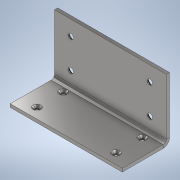
# Autodesk Inventor part: Pletina
Saved by Autodesk Inventor 2021 (Build 250183000, 183)
## iProperties
Created: 2020-10-24
Part Number: Pletina
Material: Steel, Carbon
Document SubType Name: Sheet Metal
Designer: juanj
Density: 7.85 g/cm^3
Sheet Metal Rule: Default_mm
Appearance: Semi-Polished
Author: juanj
Autodesk Inventor part; units mm, degrees
ref_plane "YZ Plane" through (0, 0, 0) normal (1, 0, 0) x (0, 1, 0)
ref_plane "XZ Plane" through (0, 0, 0) normal (0, 1, 0) x (-1, 0, 0)
ref_plane "XY Plane" through (0, 0, 0) normal (0, 0, 1) x (1, 0, 0)
sketch "Sketch1" plane through (0, 0, 0) normal (0, 1, 0) x (-1, 0, 0)
  line L0 (85, 72) -> (-85, 72)
  line L1 (-85, 72) -> (-85, 0)
  line L2 (-85, 0) -> (85, 0)
  line L3 (85, 0) -> (85, 72)
  point P0 (0, 0)
  dimension "d3" = 170
  dimension "d4" = 72
  dimension "d5" = 85
  dimension "d6" = 72
  measures "d3" distance of L2.end L1.end
  measures "d4" distance of L1.end L0.end
  measures "d5" distance from line of point (0, 0) L3
  measures "d6" distance from line of point (0, 0) L0
extrude "Plate1" add sketch "Sketch1" along normal blind 5
sketch "Sketch2" plane through (0, 5, 0) normal (0, 1, 0) x (1, 0, 0)
  line L0 (85, 0) -> (85, -72) projected
  line L1 (85, -72) -> (-85, -72) projected
  point P0 (0, 0)
  point P1 (60, -56.5)
  dimension "d43" = 90
  dimension "d8" = 25
  dimension "d9" = 15.5
  measures "d8" distance from line of L0 point (60, -56.5)
  measures "d9" distance from line of L1 point (60, -56.5)
hole "Hole1" at (60, 5, 56.5) direction (0, -1, 0) diameter 6 end through all countersink diameter 12 countersink angle 90
pattern_linear "Rectangular Pattern1" count 2 spacing 120 along (-1, 0, 0) count 2 spacing 40 along (0, 0, -1) of "Hole1"
sketch "Sketch4" plane through (-85, 0, 5) normal (0, 0, -1) x (-1, 0, 0)
  line L0 (-170, 0) -> (0, 0)
  line L1 (0, 0) -> (0, 95)
  line L2 (0, 95) -> (-170, 95)
  line L3 (-170, 95) -> (-170, 0)
  constraints: 6 end point, 1 horizontal, 1 perpendicular, 1 vertical
edge flange "Flange1" height 95 angle 90 thickness 5 bend radius 5 thickness toward (0, 0, -1) relief tear relief width 5 relief depth 2.5 edges at (0, 5, 0) wall of the first edge with corners at (85, 0, 5) (-85, 0, 5) (-85, 95, 5) (85, 95, 5)
bend "Bend1"
corner "Corner1"
sketch "Sketch7" plane through (85, 95, 0) normal (0, 0, -1) x (-1, 0, 0)
  point P0 (25, -22.502)
hole "Hole4" at (60, 72.498, 0) direction (0, 0, 1) diameter 8 end through all countersink diameter 16 countersink angle 90
pattern_linear "Rectangular Pattern6" count 2 spacing 120 along (-1, 0, 0) of "Hole4"
pattern_linear "Rectangular Pattern7" count 2 spacing 45 along (0, -1, 0) of "Hole4", "Rectangular Pattern6"
equation "\"d15\" = Thickness"
equation "\"d73\" = Thickness"
equation "\"d7\" = Thickness"
equation "\"d38\" = BendReliefWidth"
equation "\"d39\" = BendReliefDepth"
equation "\"d40\" = MinimumRemnant"
equation "\"d41\" = TransitionRadius"
equation "\"d44\" = BendRadius"
equation "\"d45\" = CornerReliefSize"
equation "\"d46\" = GapSize"
equation "\"d47\" = JacobiRadiusSize"
equation "\"BendRadius\" = Thickness"
equation "\"BendReliefWidth\" = Thickness"
equation "\"BendReliefDepth\" = 0.5 * Thickness"
equation "\"TransitionRadius\" = BendRadius"
equation "\"JacobiRadiusSize\" = BendRadius"
equation "\"GapSize\" = Thickness"
equation "\"Thickness\" = 5"
equation "\"MinimumRemnant\" = 10"
equation "\"CornerReliefSize\" = 20"
body "Solid1"
